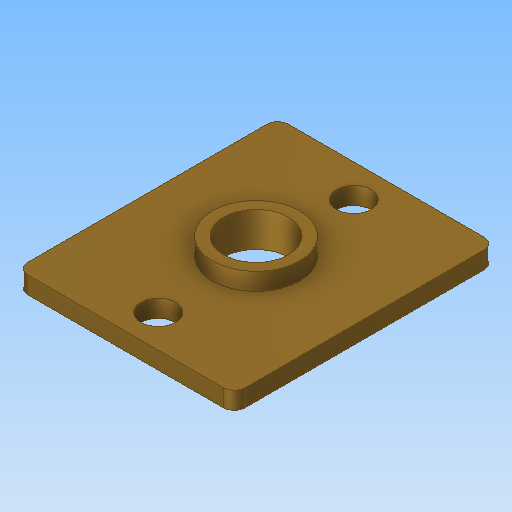
# Autodesk Inventor part: Encoder Front Plate
Saved by Autodesk Inventor 2017 SP1 (Build 210196100, 196)
## iProperties
Created: 2018-12-30
Part Number: Encoder Front Plate
Material: Brass, Soft Yellow
Document SubType Name: Modeling
Designer: Dylan Rice
Density: 8.47 g/cm^3
Appearance: Brass - Satin
Author: Dylan Rice
Autodesk Inventor part; units mm, degrees
ref_plane "YZ Plane" through (0, 0, 0) normal (1, 0, 0) x (0, 1, 0)
ref_plane "XZ Plane" through (0, 0, 0) normal (0, 1, 0) x (-1, 0, 0)
ref_plane "XY Plane" through (0, 0, 0) normal (0, 0, 1) x (1, 0, 0)
sketch "Sketch1" plane through (0, 0, 0) normal (0, 1, 0) x (-1, 0, 0)
  line L0 (-5, 6) -> (5, 6)
  line L1 (5, 6) -> (5, -6)
  line L2 (5, -6) -> (-5, -6)
  line L3 (-5, -6) -> (-5, 6)
  line L4 (-5, 6) -> (5, -6) construction
  line L5 (5, 6) -> (-5, -6) construction
  circle A0 centre (0, 0) radius 1.5
  line L6 (5, 0) -> (-5, 0) construction
  line L7 (0, 6) -> (0, -6) construction
  circle A1 centre (0, 4.5) radius 0.8
  circle A2 centre (0, -4.5) radius 0.8
  dimension "d0" = 10
  dimension "d1" = 12
  dimension "d2" = 3
  dimension "d3" = 9
  dimension "d4" = 1.6
  constraints: 16 end point, 6 midpoint, 3 centre point, 2 parallel, 2 point on line, 1 coincident, 1 horizontal, 1 perpendicular, 1 other
  measures "d0" distance between parallel lines of L3 L1
  measures "d1" distance between parallel lines of L2 L0
  measures "d2" diameter of A0
  measures "d3" distance of A2.centre A1.centre
  measures "d4" diameter of A2
extrude "Extrusion1" add sketch "Sketch1" along normal blind 0.8
fillet "Fillet1" radius 0.5 4 edges at (-5, 0.4, 6) (5, 0.4, 6) (5, 0.4, -6) (-5, 0.4, -6)
sketch "Sketch2" plane through (0, 0.8, 0) normal (0, 1, 0) x (1, 0, 0)
  circle A0 centre (0, 0) radius 1.5 projected
  circle A1 centre (0, 0) radius 2
  dimension "d9" = 4
  constraints: 1 centre point
  measures "d9" diameter of A1
extrude "Extrusion2" add sketch "Sketch2" along normal blind 0.8
body "Solid1"
